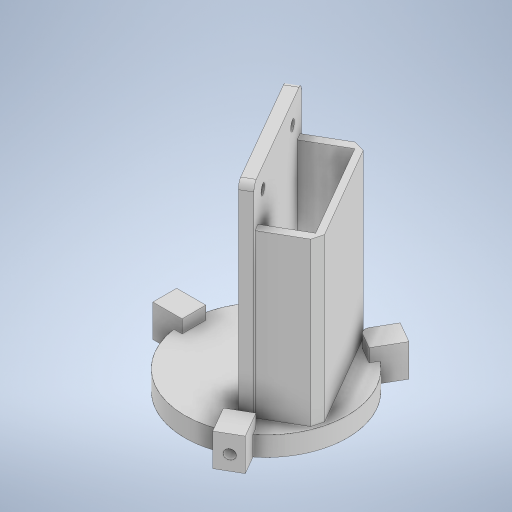
# Autodesk Inventor part: Electronic casing
Saved by Autodesk Inventor 2024 (Build 280153000, 153)
## iProperties
Created: 2024-03-27
Part Number: Electronic casing
Material: Generic
Document SubType Name: Modeling
Designer: auror
Density: 1 g/cm^3
Appearance: Default
Author: auror
Autodesk Inventor part; units mm, degrees
ref_plane "YZ Plane" through (0, 0, 0) normal (1, 0, 0) x (0, 1, 0)
ref_plane "XZ Plane" through (0, 0, 0) normal (0, 1, 0) x (-1, 0, 0)
ref_plane "XY Plane" through (0, 0, 0) normal (0, 0, 1) x (1, 0, 0)
sketch "Sketch9" plane through (0, 0, 0) normal (0, 1, 0) x (-1, 0, 0)
  line L0 (37.6236, 0) -> (-39.3749, 0) construction
  line L1 (0, 0) -> (-26.8726, 46.5447) construction
  line L2 (0, 0) -> (-26.275, -45.5096) construction
  line L3 (31.2294, 3.6686) -> (31.2294, -3.6686)
  line L4 (31.2294, 3.6686) -> (24.7294, 3.6686)
  line L5 (31.2294, -3.6686) -> (24.7294, -3.6686)
  line L6 (0, 0) -> (-18.4784, 42.9064) construction
  line L7 (0, 0) -> (-25.1787, 33.7798) construction
  line L8 (0, 0) -> (31.2294, 3.6686) construction
  line L9 (-12.4376, 28.8797) -> (-18.7918, 25.2111)
  line L10 (-12.4376, 28.8797) -> (-9.1876, 23.2506)
  line L11 (-18.7918, 25.2111) -> (-15.5418, 19.582)
  line L12 (0, 0) -> (-18.2948, -42.48) construction
  line L13 (-18.2948, -42.48) -> (0, 0) construction
  line L14 (0, 0) -> (-26.6993, -35.8199) construction
  line L15 (-18.7918, -25.2111) -> (-12.4376, -28.8797)
  line L16 (-18.7918, -25.2111) -> (-15.5418, -19.582)
  line L17 (-12.4376, -28.8797) -> (-9.1876, -23.2506)
  arc A0 (-15.5418, 19.582) -> (-15.5418, -19.582) centre (0, 0) ccw
  arc A1 (-9.1876, -23.2506) -> (24.7294, -3.6686) centre (0, 0) ccw
  arc A2 (24.7294, 3.6686) -> (-9.1876, 23.2506) centre (0, 0) ccw
  line L18 (0, 0) -> (31.2294, -3.6686) construction
  dimension "d131" = 120
  dimension "d132" = 120
  dimension "d136" = 6.7
  dimension "d137" = 6.7
  dimension "d139" = 6.7
  dimension "d140" = 6.7
  dimension "d220" = 6.5
  dimension "d221" = 6.5
  dimension "d222" = 25
  dimension "d223" = 25
  dimension "d224" = 25
  dimension "d225" = 6.5
  dimension "d227" = 6.5
  dimension "d228" = 6.5
  dimension "d236" = 6.7
  dimension "d237" = 6.7
  constraints: 38 end point, 6 point on circle, 4 perpendicular, 4 point on line, 3 centre point, 3 horizontal, 2 coincident, 1 vertical
  measures "d131" angle of L2 L0
  measures "d132" angle of L1 L0
  measures "d136" angle of L1 L6
  measures "d137" angle of L7 L1
  measures "d139" angle of L2 L12
  measures "d140" angle of L2 L14
  measures "d220" distance of L15.end L17.end
  measures "d221" distance of L9.end L11.end
  measures "d222" radius of A0
  measures "d223" radius of A1
  measures "d224" radius of A2
  measures "d225" distance of L3.end L5.end
  measures "d227" distance of L9.start L10.end
  measures "d228" distance of L15.start L16.end
  measures "d236" angle of L0 L8
  measures "d237" angle of L18 L0
extrude "Extrusion4" add sketch "Sketch9" along normal blind 6
sketch "Sketch10" plane through (18.7918, 0, 25.2111) normal (0.5, 0, 0.8660254) x (0.8660254, 0, -0.5)
  line L0 (0, 0) -> (0, 6) projected
  line L1 (-7.3372, 0) -> (0, 0) projected
  point P0 (-3.6686, 0)
  point P1 (-3.5, 4.5)
  point P2 (0, 3)
  dimension "d143" = 3.5
  dimension "d144" = 4.5
  constraints: 1 midpoint
  measures "d143" horizontal distance of point (0, 3) point (-3.5, 4.5)
  measures "d144" distance from line of L1 point (-3.5, 4.5)
hole "Hole5" at (15.7607, 4.5, 26.9611) direction (-0.5, 0, -0.8660254) diameter 3 depth 8 tip angle 118 counterbore diameter 4 counterbore depth 0
sketch "Sketch11" plane through (12.4376, 0, -28.8797) normal (0.5, 0, -0.8660254) x (-0.8660254, 0, -0.5)
  line L0 (-7.3372, 0) -> (0, 0) projected
  point P0 (-3.6686, 0)
  point P1 (-3.5001, 4.5)
  dimension "d152" = 4.5
  measures "d152" distance from line of L0 point (-3.5, 4.5)
hole "Hole6" at (15.4688, 4.5, -27.1297) direction (-0.5, 0, 0.8660254) diameter 3 depth 8 tip angle 118 counterbore diameter 4 counterbore depth 0
sketch "Sketch12" plane through (-31.2294, 0, -3.6686) normal (-1, 0, 0) x (0, 0, 1)
  line L0 (0, 0) -> (7.3372, 0) projected
  point P0 (3.6686, 0)
  point P1 (3.5, 4.5)
  dimension "d160" = 4.5
  measures "d160" distance from line of L0 point (3.5, 4.5)
hole "Hole7" at (-31.2294, 4.5, -0.1686) direction (1, 0, 0) diameter 3 depth 8 tip angle 118 counterbore diameter 4 counterbore depth 0
sketch "Sketch13" plane through (0, 6, 0) normal (0, 1, 0) x (1, 0, 0)
  line L0 (0, -31.2314) -> (0, 39.2316) construction
  line L1 (11.4285, -21.7947) -> (-13.356, 21.1333) construction
  arc A0 (9.1876, 23.2506) -> (-24.7294, 3.6686) centre (0, 0) ccw construction
  line L2 (8.9539, -17.5087) -> (11.985, -15.7587)
  line L3 (8.9539, -17.5087) -> (-11.0461, 17.1324)
  line L4 (-11.0461, 17.1324) -> (-8.015, 18.8824)
  line L5 (-8.015, 18.8824) -> (11.985, -15.7587)
  dimension "d168" = -30
  dimension "d169" = 1
  dimension "d176" = 40
  dimension "d178" = 3.5
  dimension "d238" = 3.5
  constraints: 12 end point, 2 perpendicular, 2 point on line, 1 collinear, 1 point on circle, 1 vertical
  measures "d168" angle of L0 L1
  measures "d169" distance from line of A0.centre L1
  measures "d176" distance of L3.end L2.start
  measures "d178" distance of L2.start L2.end
  measures "d238" distance of L3.end L4.end
extrude "Extrusion5" add sketch "Sketch13" along normal blind 63
sketch "Sketch14" plane through (0, 6, 0) normal (0, 1, 0) x (1, 0, 0)
  line L0 (11.985, -15.7587) -> (-8.015, 18.8824) projected
  line L1 (-8.015, 18.8824) -> (11.985, -15.7587) projected
  line L2 (1.985, 1.5618) -> (17.122, 10.3012) construction
  line L3 (21.4933, -6.2276) -> (4.9933, 22.3513)
  line L4 (4.9933, 22.3513) -> (-6.265, 15.8513)
  line L5 (21.4933, -6.2276) -> (10.235, -12.7276)
  line L6 (3.2718, 24.1641) -> (98.9629, -140.4088) construction
  line L7 (10.235, -12.7276) -> (26.8444, -3.1382) construction
  line L8 (-6.265, 15.8513) -> (10.0933, 25.2005) construction
  line L9 (22.3158, -8.5884) -> (11.4629, -14.8543)
  line L10 (3.2718, 24.1641) -> (-7.4803, 17.9563)
  line L11 (23.2254, -5.2276) -> (6.6704, 23.2443)
  line L12 (3.2718, 24.1641) -> (6.6704, 23.2443)
  line L13 (23.2254, -5.2276) -> (22.3158, -8.5884)
  point P0 (0, 0)
  point P1 (10.235, -12.7276)
  point P2 (11.4629, -14.8543)
  point P3 (-7.4803, 17.9563)
  point P4 (-6.265, 15.8513)
  dimension "d181" = 13
  dimension "d182" = 13
  dimension "d184" = 20
  dimension "d185" = 16.5
  dimension "d186" = 33
  dimension "d192" = 2.5
  dimension "d193" = 2.5
  dimension "d194" = 2
  dimension "d195" = 1.9
  constraints: 24 end point, 9 point on line, 6 perpendicular, 2 coincident, 1 midpoint, 1 parallel
  measures "d181" distance from line of L0 L3.start
  measures "d182" distance from line of L0 L3.end
  measures "d184" distance of point (11.985, -15.759) L2.start
  measures "d185" distance from line of L2 L3.start
  measures "d186" distance of L3.end L3.start
  measures "d192" distance of L3.start L9.start
  measures "d193" distance of L6.start L3.end
  measures "d194" distance of L3.start L11.start
  measures "d195" distance of L3.end L11.end
extrude "Extrusion6" add sketch "Sketch14" along normal blind 50 contours L0 L5 L3 L4 L10 L12 L11 L13 L9
sketch "Sketch15" plane through (8.9539, 6, 17.5087) normal (-0.8660254, 0, 0.5) x (0.5, 0, 0.8660254)
  line L0 (-40, 63) -> (0, 63) projected
  line L1 (-40, 0) -> (-40, 63) projected
  point P0 (-19.6399, -6)
  point P1 (-32.5, 56.6)
  point P2 (-7.5, 56.6)
  point P3 (-7.5, 11.4)
  point P4 (-32.5, 11.4)
  dimension "d201" = 0
  dimension "d202" = 25
  dimension "d203" = 0
  dimension "d204" = 45.2
  dimension "d205" = 0
  dimension "d206" = 25
  dimension "d209" = 6.4
  dimension "d210" = 7.5
  measures "d201" vertical distance of point (-7.5, 56.6) point (-32.5, 56.6)
  measures "d202" distance of point (-7.5, 56.6) point (-32.5, 56.6)
  measures "d203" horizontal distance of point (-7.5, 11.4) point (-7.5, 56.6)
  measures "d204" distance of point (-7.5, 56.6) point (-7.5, 11.4)
  measures "d205" vertical distance of point (-32.5, 11.4) point (-7.5, 11.4)
  measures "d206" distance of point (-7.5, 11.4) point (-32.5, 11.4)
  measures "d209" distance from line of L0 point (-32.5, 56.6)
  measures "d210" distance from line of L1 point (-32.5, 56.6)
hole "Hole8" at (-7.2961, 62.6, -10.6372) at (5.2039, 62.6, 11.0135) at (5.2039, 17.4, 11.0135) at (-7.2961, 17.4, -10.6372) direction (0.8660254, 0, -0.5) diameter 3 depth 15 tip angle 118 counterbore diameter 4 counterbore depth 0
fillet "Fillet3" radius 2 1 edges at (-9.5305, 69, -18.0074)
fillet "Fillet4" radius 2 1 edges at (10.4695, 69, 16.6337)
sketch "Sketch16" plane through (0, 6, 0) normal (0, 1, 0) x (1, 0, 0)
  line L0 (12.4376, -28.8797) -> (18.7918, -25.2111)
  line L1 (12.4376, -28.8797) -> (7.9376, -21.0855)
  line L2 (7.9376, -21.0855) -> (14.2918, -17.4169)
  line L3 (14.2918, -17.4169) -> (18.7918, -25.2111)
  line L4 (18.7918, -25.2111) -> (15.5418, -19.582) projected
  point P0 (0, 0)
  dimension "d231" = 180
  dimension "d232" = 0
  dimension "d240" = 9
  constraints: 8 end point, 2 perpendicular
  measures "d231" angle of L4 L3
  measures "d232" distance of L0.end L3.end
  measures "d240" distance of L0.start L1.end
extrude "Extrusion7" add sketch "Sketch16" along normal blind 4
pattern_circular "Circular Pattern1" count 3 over 360 about axis through (0, -10, 0) along (0, 1, 0) of "Extrusion7"
fillet "Fillet5" radius 2 1 edges at (7.9376, 8, -21.0855)
body "Solid2"
